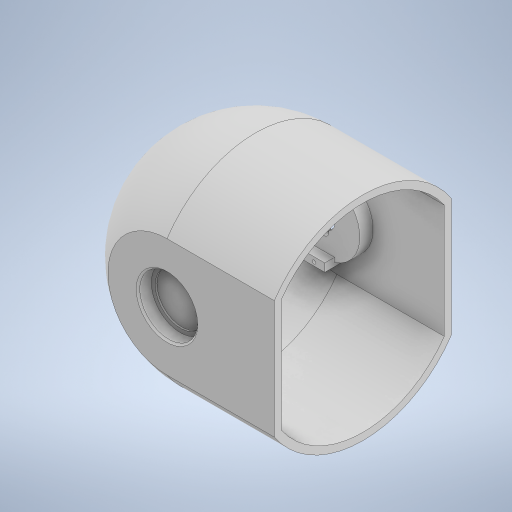
# Autodesk Inventor part: 메인 상단 헤드
Saved by Autodesk Inventor 2023 (Build 270158000, 158)
## iProperties
Created: 2022-06-06
Part Number: 메인 상단 헤드
Material: 일반
Document SubType Name: Modeling
Designer: fly01
Density: 1 g/cm^3
Appearance: 기본값
Author: fly01
Autodesk Inventor part; units mm, degrees
ref_plane "YZ Plane" through (0, 0, 0) normal (1, 0, 0) x (0, 1, 0)
ref_plane "XZ Plane" through (0, 0, 0) normal (0, 1, 0) x (-1, 0, 0)
ref_plane "XY Plane" through (0, 0, 0) normal (0, 0, 1) x (1, 0, 0)
sketch "스케치1" plane through (0, 0, 0) normal (0, 0, 1) x (1, 0, 0)
  circle A0 centre (0, 0) radius 59.5
  line L0 (0, 59.5) -> (0, -59.5)
  dimension "d0" = 119
  constraints: 2 end point, 2 point on circle, 1 centre point, 1 coincident, 1 vertical
  measures "d0" diameter of A0
sketch "스케치1 outline for 회전1" plane through (0, 0, 0) normal (0, 0, 1) x (1, 0, 0)
  line L0 (0, 59.5) -> (0, -59.5)
  arc A0 (0, -59.5) -> (0, 59.5) centre (0, 0) ccw
revolve "회전1" add sketch "스케치1 outline for 회전1" angle 360 about axis through (0, 59.5, 0) along (0, -1, 0)
sketch "스케치2" plane through (0, 0, 0) normal (1, 0, 0) x (0, 1, 0)
  line L0 (-88.471699, 49.5) -> (88.471699, 49.5)
  line L1 (88.471699, 49.5) -> (88.471699, -49.5)
  line L2 (88.471699, -49.5) -> (-88.471699, -49.5)
  line L3 (-88.471699, -49.5) -> (-88.471699, 49.5)
  line L4 (-88.471699, 49.5) -> (88.471699, -49.5) construction
  line L5 (88.471699, 49.5) -> (-88.471699, -49.5) construction
  line L6 (-88.471699, 113.085262) -> (88.471699, 113.085262)
  line L7 (88.471699, 113.085262) -> (88.471699, -113.085262)
  line L8 (88.471699, -113.085262) -> (-88.471699, -113.085262)
  line L9 (-88.471699, -113.085262) -> (-88.471699, 113.085262)
  line L10 (-88.471699, 113.085262) -> (88.471699, -113.085262) construction
  line L11 (88.471699, 113.085262) -> (-88.471699, -113.085262) construction
  point P0 (0, 0)
  dimension "d2" = 99
  constraints: 24 end point, 4 midpoint, 4 parallel, 2 horizontal, 2 perpendicular
  measures "d2" distance of L0.end L1.end
sketch "스케치2 outline for 돌출1" plane through (0, 0, 0) normal (1, 0, 0) x (0, 1, 0)
  line L0 (88.471699, 113.085262) -> (-88.471699, 113.085262)
  line L1 (88.471699, 49.5) -> (88.471699, 113.085262)
  line L2 (-88.471699, 49.5) -> (88.471699, 49.5)
  line L3 (-88.471699, 113.085262) -> (-88.471699, 49.5)
  line L4 (-88.471699, -113.085262) -> (88.471699, -113.085262)
  line L5 (-88.471699, -49.5) -> (-88.471699, -113.085262)
  line L6 (88.471699, -49.5) -> (-88.471699, -49.5)
  line L7 (88.471699, -113.085262) -> (88.471699, -49.5)
extrude "돌출1" cut sketch "스케치2 outline for 돌출1" along normal mid plane 212.75
sketch "스케치3" plane through (0, 0, 0) normal (1, 0, 0) x (0, 1, 0)
  line L0 (-33.015148, 49.5) -> (33.015148, 49.5)
  line L1 (33.015148, -49.5) -> (-33.015148, -49.5)
  arc A0 (-33.015148, 49.5) -> (33.015148, 49.5) centre (0, 0) ccw
sketch "스케치3 outline for 돌출2" plane through (0, 0, 0) normal (1, 0, 0) x (0, 1, 0)
  line L0 (33.015148, 49.5) -> (-33.015148, 49.5)
  arc A0 (33.015148, -49.5) -> (33.015148, 49.5) centre (0, 0) ccw
  line L1 (-33.015148, -49.5) -> (33.015148, -49.5)
  arc A1 (-33.015148, 49.5) -> (-33.015148, -49.5) centre (0, 0) ccw
extrude "돌출2" add sketch "스케치3 outline for 돌출2" along normal blind 60
sketch "스케치5" plane through (0, -33.015148, 49.5) normal (0, 0, 1) x (1, 0, 0)
  circle A0 centre (0, 33.015148) radius 16.2
  dimension "d10" = 32.4
  constraints: 1 centre point, 1 coincident
  measures "d10" diameter of A0
sketch "스케치5 outline for 돌출4" plane through (0, -33.015148, 49.5) normal (0, 0, 1) x (1, 0, 0)
  circle A0 centre (0, 33.015148) radius 16.2
extrude "돌출4" cut sketch "스케치5 outline for 돌출4" against normal blind 7.4
mirror "미러1" about plane through (0, 0, 0) normal (0, 0, 1) of "돌출4"
chamfer "모따기2" distance 1 angle 45 2 edges at (-16.2, 0, 49.5) (-16.2, 0, -49.5)
shell "쉘1" thickness 4 removed faces 1 at (60, 18.496646, 1.76927)
sketch "스케치7" plane through (0, 0, -42.1) normal (0, 0, -1) x (-1, 0, 0)
  circle A0 centre (0, 0) radius 3.85
  dimension "d20" = 7.7
  constraints: 1 centre point, 1 coincident
  measures "d20" diameter of A0
sketch "스케치7 outline for 돌출5" plane through (0, 0, -42.1) normal (0, 0, -1) x (-1, 0, 0)
  circle A0 centre (0, 0) radius 3.85
extrude "돌출5" cut sketch "스케치7 outline for 돌출5" against normal blind 12
sketch "스케치8" plane through (0, 0, -38.1) normal (0, 0, 1) x (1, 0, 0)
  circle A0 centre (0, 0) radius 3.85 projected
  circle A1 centre (0, 0) radius 6.25
  circle A2 centre (0, -6.25) radius 3
  point P0 (2.912319, -5.53)
  point P1 (-2.912319, -5.53)
  dimension "d23" = 12.5
  dimension "d24" = 6
  constraints: 1 centre point, 1 coincident, 3 other
  measures "d24" diameter of A2
sketch "스케치8 outline for 돌출6" plane through (0, 0, -38.1) normal (0, 0, 1) x (1, 0, 0)
  arc A0 (2.912319, -5.53) -> (-2.912319, -5.53) centre (0, 0) ccw
  arc A1 (-2.912319, -5.53) -> (2.912319, -5.53) centre (0, -6.25) ccw
  circle A2 centre (0, 0) radius 3.85
extrude "돌출6" cut sketch "스케치8 outline for 돌출6" against normal blind 8.25
sketch "스케치10" plane through (0, 0, -38.1) normal (0, 0, 1) x (1, 0, 0)
  line L0 (0, 0) -> (0, -16.8) construction
  line L1 (0, 0) -> (0, 6.3) construction
  line L2 (-6, 6.3) -> (6, 6.3)
  line L3 (6, 6.3) -> (6, -16.8)
  line L4 (6, -16.8) -> (-6, -16.8)
  line L5 (-6, -16.8) -> (-6, 6.3)
  line L6 (-6, -5.25) -> (0, -5.25) construction
  line L7 (-6, -21.35) -> (6, -21.35)
  line L8 (6, -21.35) -> (6, 10.85)
  line L9 (6, 10.85) -> (-6, 10.85)
  line L10 (-6, 10.85) -> (-6, -21.35)
  line L11 (-6, -21.35) -> (6, 10.85) construction
  line L12 (6, -21.35) -> (-6, 10.85) construction
  line L13 (0, -5.25) -> (0, 8.85)
  circle A0 centre (0, 8.85) radius 1
  circle A1 centre (0, -19.35) radius 1
  arc A2 (-2.904738, -5.25) -> (2.904738, -5.25) centre (0, -6) ccw
  arc A3 (2.904738, -5.25) -> (-2.904738, -5.25) centre (0, 0) ccw
  circle A4 centre (0, 0) radius 3.85
  point P0 (-6, -16.8)
  point P1 (6, 6.3)
  point P2 (-6, 6.3)
  dimension "d28" = 6.3
  dimension "d29" = 12
  dimension "d30" = 32.2
  dimension "d31" = 14.1
  dimension "d32" = 2
  constraints: 28 end point, 5 midpoint, 4 parallel, 3 perpendicular, 3 vertical, 2 centre point, 2 horizontal, 1 coincident, 1 point on line, 1 symmetric about line, 1 other
  measures "d28" distance of L1.end L0.start
  measures "d29" distance of L2.start L2.end
  measures "d30" distance of L7.end L8.end
  measures "d31" distance of L6.end L13.end
  measures "d32" diameter of A0
sketch "스케치10 outline for 돌출7" plane through (0, 0, -38.1) normal (0, 0, 1) x (1, 0, 0)
  line L0 (-6, -21.35) -> (6, -21.35)
  line L1 (-6, -16.8) -> (-6, -21.35)
  line L2 (6, -21.35) -> (6, -16.8)
  line L3 (6, -16.8) -> (-6, -16.8)
  circle A0 centre (0, -19.35) radius 1
  line L4 (-6, 6.3) -> (6, 6.3)
  line L5 (-6, 10.85) -> (-6, 6.3)
  line L6 (6, 6.3) -> (6, 10.85)
  line L7 (6, 10.85) -> (-6, 10.85)
  circle A1 centre (0, 8.85) radius 1
extrude "돌출7" add sketch "스케치10 outline for 돌출7" along normal blind 5.4
sketch "스케치11" plane through (0, 0, -42.1) normal (0, 0, -1) x (-1, 0, 0)
  circle A0 centre (0, 0) radius 3.85 projected
  circle A1 centre (0, 0) radius 14
  dimension "d35" = 28
  constraints: 1 centre point, 1 coincident
  measures "d35" diameter of A1
sketch "스케치11 outline for 돌출8" plane through (0, 0, -42.1) normal (0, 0, -1) x (-1, 0, 0)
  circle A0 centre (0, 0) radius 14
extrude "돌출8" cut sketch "스케치11 outline for 돌출8" against normal blind 1
mirror "미러2" about plane through (0, 0, 0) normal (0, 0, 1) of "돌출8"
sketch "스케치10 outline for 돌출9" plane through (0, 0, -38.1) normal (0, 0, 1) x (1, 0, 0)
  line L0 (-6, -21.35) -> (6, -21.35)
  line L1 (-6, -16.8) -> (-6, -21.35)
  line L2 (6, -21.35) -> (6, -16.8)
  line L3 (6, -16.8) -> (-6, -16.8)
  circle A0 centre (0, -19.35) radius 1
extrude "돌출9" add sketch "스케치10 outline for 돌출9" against normal up to surface (7.4 mm away)
